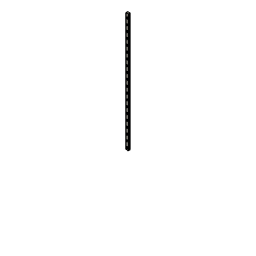
MGN7 Rail - 300mm (Autodesk Fusion 360 design; units mm, degrees)
Autodesk Fusion 360 part; units mm, degrees
sketch "Rail Profile" plane through (0, 0, 0) normal (0, 0, 1) x (1, 0, 0)
  arc A0 (-3.1262, 2.1009) -> (-3.4118, 2.3379) centre (-3.7, 1.7) ccw
  arc A1 (-3.1262, 2.1009) -> (-3.0163, 2.0374) centre (-3.0032, 2.1868) ccw
  line L0 (-3.0163, 2.0374) -> (-2.5869, 1.9998)
  arc A2 (-2.45, 1.8504) -> (-2.5869, 1.9998) centre (-2.6, 1.8504) ccw
  line L1 (-2.45, 1.8504) -> (-2.45, 1.5496)
  arc A3 (-2.5869, 1.4002) -> (-2.45, 1.5496) centre (-2.6, 1.5496) ccw
  line L2 (-2.5869, 1.4002) -> (-3.0163, 1.3626)
  arc A4 (-3.0163, 1.3626) -> (-3.1262, 1.2991) centre (-3.0032, 1.2132) ccw
  arc A5 (-3.4118, 1.0621) -> (-3.1262, 1.2991) centre (-3.7, 1.7) ccw
  arc A6 (-3.4118, 1.0621) -> (-3.5, 0.9254) centre (-3.35, 0.9254) ccw
  line L3 (-3.5, 0.9254) -> (-3.5, 0.3)
  line L4 (-3.5, 0.3) -> (-3.2, 0)
  line L5 (-3.2, 0) -> (3.2, 0)
  line L6 (3.2, 0) -> (3.5, 0.3)
  line L7 (3.5, 0.3) -> (3.5, 0.9254)
  arc A7 (3.5, 0.9254) -> (3.4118, 1.0621) centre (3.35, 0.9254) ccw
  arc A8 (3.1262, 1.2991) -> (3.4118, 1.0621) centre (3.7, 1.7) ccw
  arc A9 (3.1262, 1.2991) -> (3.0163, 1.3626) centre (3.0032, 1.2132) ccw
  line L8 (3.0163, 1.3626) -> (2.5869, 1.4002)
  arc A10 (2.45, 1.5496) -> (2.5869, 1.4002) centre (2.6, 1.5496) ccw
  line L9 (2.45, 1.5496) -> (2.45, 1.8504)
  arc A11 (2.5869, 1.9998) -> (2.45, 1.8504) centre (2.6, 1.8504) ccw
  line L10 (2.5869, 1.9998) -> (3.0163, 2.0374)
  arc A12 (3.0163, 2.0374) -> (3.1262, 2.1009) centre (3.0032, 2.1868) ccw
  arc A13 (3.4118, 2.3379) -> (3.1262, 2.1009) centre (3.7, 1.7) ccw
  arc A14 (3.4118, 2.3379) -> (3.5, 2.4746) centre (3.35, 2.4746) ccw
  line L11 (3.5, 2.4746) -> (3.5, 4.4)
  line L12 (3.5, 4.4) -> (3.1, 4.8)
  line L13 (3.1, 4.8) -> (-3.1, 4.8)
  line L14 (-3.1, 4.8) -> (-3.5, 4.4)
  line L15 (-3.5, 4.4) -> (-3.5, 2.4746)
  arc A15 (-3.5, 2.4746) -> (-3.4118, 2.3379) centre (-3.35, 2.4746) ccw
  constraint midpoint origin L5
extrude "Extrude1" add sketch "Rail Profile" along normal blind 300 contours A0 A1 L0 A2 L1 A3 L2 A4 A5 A6 L3 L4 L5 L6 L7 A7 A8 A9 L8 A10 L9 A11 L10 A12 A13 A14 L11 L12 L13 L14 L15 A15
sketch "Screw Hole Profile" plane through (0, 0, 0) normal (0, 1, 0) x (1, 0, 0)
  line L0 (0, 0) -> (0, -5) construction
  circle A0 centre (0, -5) radius 2.1
  circle A1 centre (0, -5) radius 1.2
  dimension "d4" = 5
  dimension "d5" = 4.2
  dimension "d6" = 2.4
  constraint coincident L0.start origin
  constraint vertical L0
  constraint coincident L0.end A0.centre
  constraint concentric A0 A1
  measures "d4" distance of L0.start L0.end
  measures "d5" diameter of A0
  measures "d6" diameter of A1
extrude "Extrude2" cut sketch "Screw Hole Profile" along normal up to surface (4.8 mm away) contours A1
extrude "Extrude3" cut sketch "Screw Hole Profile" along normal blind 2.3
chamfer "Chamfer1" distance 0.4 angle 45 2 edges at (-1.9579, 0, 5.7594) (-1.1188, 4.8, 4.5661)
pattern_linear "R-Pattern1" count 50 spacing 15 along (0, 0, 1) of "Extrude2", "Extrude3", "Chamfer1"
equation "d2 = RailLength"
equation "RailLength = 300 mm" comment "Length of the linear rail"
